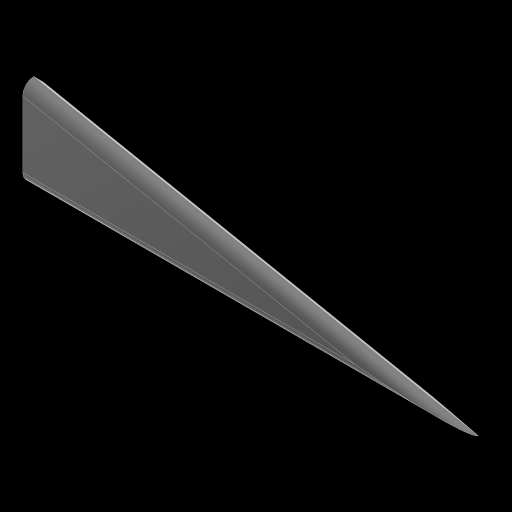
# Autodesk Inventor part: WedgeUHMWPiece
Saved by Autodesk Inventor 2024.2 (Build 282272000, 272)
## iProperties
Created: 2021-02-16
Part Number: WedgeUHMWPiece
Material: Custom TPU
Document SubType Name: Modeling
Designer: Esketitttttt
Density: 1.21 g/cm^3
Appearance: Smooth - Black
Mass: 12.5604 g
Surface Area: 51.0856 cm^2
Volume: 10.3805 cm^3
Author: Esketitttttt
Autodesk Inventor part; units mm, degrees
ref_plane "YZ Plane" through (0, 0, 0) normal (1, 0, 0) x (0, 1, 0)
ref_plane "XZ Plane" through (0, 0, 0) normal (0, 1, 0) x (-1, 0, 0)
ref_plane "XY Plane" through (0, 0, 0) normal (0, 0, 1) x (1, 0, 0)
sketch "Sketch1" plane through (0, 0, 0) normal (0, 0, 1) x (1, 0, 0)
  line L0 (0, 0) -> (0, 25.4)
  line L1 (0, 25.4) -> (127, 0)
  line L2 (0, 25.4) -> (129.5151, 25.4) construction
  line L3 (127, 0) -> (0, 0)
  line L4 (62.8712, 6.35) -> (6.35, 17.6542)
  line L5 (6.35, 17.6542) -> (6.35, 6.35)
  line L6 (6.35, 6.35) -> (62.8712, 6.35)
  line L7 (13.97, 6.35) -> (13.97, 16.1302)
  dimension "d0" = 25.4
  dimension "d35" = 127
  dimension "d41" = 6.35
  dimension "d42" = 13.97
  constraints: 16 end point, 2 horizontal, 2 point on line, 1 equal length, 1 parallel, 1 vertical, 2 other
  measures "d0" distance of L0.start L0.end
  measures "d35" distance of L1.end L0.start
  measures "d41" distance between parallel lines of L1 L4
  measures "d42" distance between parallel lines of L0 L7
extrude "Extrusion1" add sketch "Sketch1" along normal blind 6.35 contours L0 L1 L3 | L6 L7 L4 | L7 L6 L5 L4
sketch "Sketch2" plane through (0, 0, 0) normal (-1, 0, 0) x (0, 0, 1)
  line L0 (0, 25.4) -> (0, 0) construction
  line L1 (0, 0) -> (6.35, 0) construction
  line L2 (3.175, 0) -> (3.175, 8.4667) construction
  line L3 (3.175, 8.4667) -> (3.175, 16.9333) construction
  dimension "d4" = 25.4
  dimension "d6" = 8.4667
  dimension "d25" = 8.4667
  constraints: 4 end point, 2 coincident, 1 midpoint, 1 point on line, 1 vertical
  measures "d4" distance of L0.start L0.end
  measures "d6" distance of L2.end L3.end
  measures "d25" vertical distance of L0.start point (3.175, 16.933)
hole "Hole1" at (0, 8.4667, 3.175) at (0, 16.9333, 3.175) direction (1, 0, 0) diameter 2.794 depth 7.62 tip angle 118
sketch "Sketch3" plane through (0, 25.4, 6.35) normal (0.1961, 0.9806, 0) x (0.9806, -0.1961, 0)
  line L0 (129.5151, 0) -> (0, 0) construction
  line L1 (0, 6.35) -> (0, 0) construction
  line L2 (0, 3.175) -> (43.1717, 3.175) construction
  line L3 (9.1325, 4.572) -> (1.6604, 4.572) construction
  line L4 (0, 3.175) -> (43.1717, 3.175) construction
  line L5 (43.1717, 3.175) -> (75.5505, 3.175) construction
  point P0 (4.9813, 6.35)
  dimension "d14" = 129.5151
  dimension "d15" = 43.1717
  dimension "d17" = 32.3788
  dimension "d26" = 40
  constraints: 6 end point, 2 coincident, 2 horizontal, 1 collinear, 1 midpoint, 1 parallel
  measures "d14" distance of L0.start L0.end
  measures "d15" distance of L2.start L2.end
  measures "d17" distance of L4.end L5.end
hole "Hole2" [suppressed]
chamfer "Chamfer1" distance 3.175 angle 45 1 edges at (63.5, 12.7, 0)
fillet "Fillet1" radius 3.175 2 edges at (63.5, 12.7, 6.35) (63.5, 0, 6.35)
fillet "Fillet1" radius 1.27 2 edges at (55.4053, 11.0811, 0) (55.4053, 0, 0)
equation "\"d25\" = 0.333333 * d4"
equation "\"d7\" = ThreadingScrew"
equation "\"d15\" = 0.333333 * d14"
equation "\"d17\" = 0.25 * d14"
equation "\"ThreadingScrew\" = 2.794"
body "Solid1"
